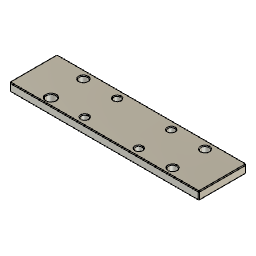
X motor reinforcement plate (Autodesk Fusion 360 design; units mm, degrees)
Autodesk Fusion 360 part; units mm, degrees
sketch "Top" plane through (0, 0, 0) normal (0, 0, 1) x (1, 0, 0)
  line L0 (-70, 0) -> (70, 0)
  line L1 (70, 0) -> (70, 35)
  line L2 (70, 35) -> (-70, 35)
  line L3 (-70, 35) -> (-70, 0)
  line L4 (-45, 29.5) -> (45, 29.5) construction
  line L5 (45, 29.5) -> (45, 5.5) construction
  line L6 (45, 5.5) -> (-45, 5.5) construction
  line L7 (-45, 5.5) -> (-45, 29.5) construction
  line L8 (70, 24.75) -> (45, 24.75) construction
  line L9 (-70, 24.75) -> (-45, 24.75) construction
  line L10 (20, 35) -> (20, 29.5) construction
  line L11 (9.991, 5.5) -> (9.991, 0) construction
  line L12 (-20, 29.5) -> (20, 29.5) construction
  line L13 (20, 29.5) -> (20, 5.5) construction
  line L14 (20, 5.5) -> (-20, 5.5) construction
  line L15 (-20, 5.5) -> (-20, 29.5) construction
  line L16 (20, 14.3708) -> (45, 14.3708) construction
  line L17 (-20, 14.3708) -> (-45, 14.3708) construction
  circle A0 centre (-45, 29.5) radius 3
  circle A1 centre (-45, 5.5) radius 3.5
  circle A2 centre (45, 29.5) radius 3
  circle A3 centre (45, 5.5) radius 3
  circle A4 centre (20, 29.5) radius 2.5
  circle A5 centre (-20, 29.5) radius 2.5
  circle A6 centre (20, 5.5) radius 2.5
  circle A7 centre (-20, 5.5) radius 2.5
  dimension "d1" = 140
  dimension "d2" = 35
  dimension "d3" = 70
  dimension "d4" = 90
  dimension "d5" = 24
  dimension "d6" = 40
  dimension "d7" = 6
  dimension "d8" = 7
  dimension "d9" = 6
  dimension "d10" = 6
  dimension "d11" = 5
  dimension "d13" = 5
  dimension "d15" = 35
  dimension "d16" = 40
  dimension "d18" = 24
  dimension "d19" = 5
  dimension "d20" = 5
  constraint horizontal L0
  constraint vertical L1
  constraint horizontal L2
  constraint vertical L3
  constraint horizontal L4
  constraint vertical L5
  constraint horizontal L6
  constraint vertical L7
  constraint coincident L1 L8.start
  constraint coincident L5 L8.end
  constraint perpendicular L5 L8
  constraint coincident L3 L9.start
  constraint coincident L7 L9.end
  constraint perpendicular L7 L9
  constraint equal L8 L9
  constraint coincident L2 L10.start
  constraint coincident L4 L10.end
  constraint perpendicular L4 L10
  constraint coincident L6 L11.start
  constraint coincident L0 L11.end
  constraint perpendicular L0 L11
  constraint equal L10 L11
  constraint horizontal L12
  constraint vertical L13
  constraint horizontal L14
  constraint vertical L15
  constraint coincident L4 L12.start
  constraint coincident L13 L16.start
  constraint coincident L5 L16.end
  constraint perpendicular L5 L16
  constraint coincident L15 L17.start
  constraint coincident L7 L17.end
  constraint perpendicular L7 L17
  constraint equal L16 L17
  constraint coincident L4.start L7.end
  constraint coincident L6.end L7.start
  constraint coincident L4.end L5.start
  constraint coincident L5.end L6.start
  constraint coincident L10.end L12.end
  constraint coincident L12.start L15.end
  constraint coincident L13.end L14.start
  constraint coincident L14.end L15.start
  measures "d1" distance of L0.start L0.end
  measures "d2" distance of L0.start L2.end
  measures "d3" distance of origin L1
  measures "d4" distance of L4.start L4.end
  measures "d5" distance of L4.start L6.end
  measures "d6" distance of L12.start L10.end
  measures "d7" diameter of A0
  measures "d8" diameter of A1
  measures "d9" diameter of A2
  measures "d10" diameter of A3
  measures "d11" diameter of A4
  measures "d13" diameter of A5
  measures "d15" distance of origin L2
  measures "d16" distance of L10.end L12.start
  measures "d18" distance of L10.end L13.end
  measures "d19" diameter of A6
  measures "d20" diameter of A7
extrude "Extrude1" add sketch "Top" along normal blind 6
chamfer "Chamfer1" distance 0.5 angle 45 15 edges at (0, 35, 0) (-70, 17.5, 0) (0, 0, 0) (70, 17.5, 0) (70, 35, 3) (-70, 35, 3) (-70, 0, 3) (-47.797, 30.5848, 0) (-48.2631, 6.7657, 0) (-22.3308, 6.404, 0) (-22.3308, 30.404, 0) (17.6692, 30.404, 0) (17.6692, 6.404, 0) (42.203, 6.5848, 0) (42.203, 30.5848, 0)
chamfer "Chamfer2" distance 0.5 angle 45 11 edges at (0.25, 0, 6) (70, 0, 3.25) (70, 17.25, 6) (42.203, 30.5848, 6) (42.203, 6.5848, 6) (17.6692, 6.404, 6) (17.6692, 30.404, 6) (-22.3308, 30.404, 6) (-22.3308, 6.404, 6) (-48.2631, 6.7657, 6) (-47.797, 30.5848, 6)
named bodies: "Plate"
